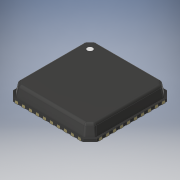
# Autodesk Inventor part: Semiconductor_QFN24-4x4
Saved by Autodesk Inventor 2018 (Build 220112000, 112)
## iProperties
Created: 2016-07-11
Part Number: Semiconductor_QFN24-4x4
Material: ABS Plastic
Document SubType Name: Modeling
Designer: Bradley
Density: 1.06 g/cm^3
Appearance: Smooth - Black
Author: Bradley
Autodesk Inventor part; units mm, degrees
ref_plane "YZ Plane" through (0, 0, 0) normal (1, 0, 0) x (0, 1, 0)
ref_plane "XZ Plane" through (0, 0, 0) normal (0, 1, 0) x (-1, 0, 0)
ref_plane "XY Plane" through (0, 0, 0) normal (0, 0, 1) x (1, 0, 0)
sketch "Sketch1" plane through (0, 0, 0) normal (0, 1, 0) x (-1, 0, 0)
  line L0 (-2.5, 3) -> (2.5, 3)
  line L1 (3, 2.5) -> (3, -2.5)
  line L2 (2.5, -3) -> (-2.5, -3)
  line L3 (-3, -2.5) -> (-3, 2.5)
  line L4 (-3, 3) -> (3, -3) construction
  line L5 (3, 3) -> (-3, -3) construction
  line L6 (3, 2.5) -> (2.5, 3)
  line L7 (-2.5, 3) -> (-3, 2.5)
  line L8 (-3, -2.5) -> (-2.5, -3)
  line L9 (2.5, -3) -> (3, -2.5)
  point P0 (0, 0)
  dimension "d0" = 6
  dimension "d1" = 6
  dimension "d68" = 0.5
  constraints: 20 end point, 8 point on line, 7 perpendicular, 2 midpoint, 2 parallel, 1 horizontal, 1 horizontal alignment
  measures "d0" distance of L4.end L5.end
  measures "d1" distance of L5.start L4.end
  measures "d68" distance of L1.start L5.start
extrude "Extrusion1" add sketch "Sketch1" along normal mid plane 0.2
sketch "Sketch2" plane through (0, -0.1, 0) normal (0, -1, 0) x (1, 0, 0)
  line L0 (2.05, 2.05) -> (-2.05, 2.05)
  line L1 (-2.05, 2.05) -> (-2.05, -2.05)
  line L2 (-2.05, -2.05) -> (2.05, -2.05)
  line L3 (2.05, -2.05) -> (2.05, 2.05)
  line L4 (2.05, 2.05) -> (-2.05, -2.05) construction
  line L5 (-2.05, 2.05) -> (2.05, -2.05) construction
  line L6 (2.5, 3) -> (-2.5, 3) projected
  line L7 (-3, 2.5) -> (-3, -2.5) projected
  line L8 (-2.5, -3) -> (2.5, -3) projected
  line L9 (3, -2.5) -> (3, 2.5) projected
  line L10 (2.375, -3) -> (2.125, -3)
  line L11 (2.125, -3) -> (2.125, -2.6)
  line L12 (2.125, -2.6) -> (2.375, -2.6)
  line L13 (2.375, -2.6) -> (2.375, -3)
  line L14 (3, -2.375) -> (2.6, -2.375)
  line L15 (2.6, -2.375) -> (2.6, -2.125)
  line L16 (2.6, -2.125) -> (3, -2.125)
  line L17 (3, -2.125) -> (3, -2.375)
  line L18 (2.375, 3) -> (2.125, 3)
  line L19 (2.125, 3) -> (2.125, 2.6)
  line L20 (2.125, 2.6) -> (2.375, 2.6)
  line L21 (2.375, 2.6) -> (2.375, 3)
  line L22 (-3, -2.375) -> (-2.6, -2.375)
  line L23 (-2.6, -2.375) -> (-2.6, -2.125)
  line L24 (-2.6, -2.125) -> (-3, -2.125)
  line L25 (-3, -2.125) -> (-3, -2.375)
  line L26 (3, -1.875) -> (2.6, -1.875)
  line L27 (2.6, -1.875) -> (2.6, -1.625)
  line L28 (2.6, -1.625) -> (3, -1.625)
  line L29 (3, -1.625) -> (3, -1.875)
  line L30 (-3, -1.875) -> (-2.6, -1.875)
  line L31 (-3, -1.625) -> (-3, -1.875)
  line L32 (-2.6, -1.625) -> (-3, -1.625)
  line L33 (-2.6, -1.875) -> (-2.6, -1.625)
  line L34 (3, -1.375) -> (2.6, -1.375)
  line L35 (2.6, -1.375) -> (2.6, -1.125)
  line L36 (2.6, -1.125) -> (3, -1.125)
  line L37 (3, -1.125) -> (3, -1.375)
  line L38 (-3, -1.375) -> (-2.6, -1.375)
  line L39 (-3, -1.125) -> (-3, -1.375)
  line L40 (-2.6, -1.125) -> (-3, -1.125)
  line L41 (-2.6, -1.375) -> (-2.6, -1.125)
  line L42 (3, -0.875) -> (2.6, -0.875)
  line L43 (2.6, -0.875) -> (2.6, -0.625)
  line L44 (2.6, -0.625) -> (3, -0.625)
  line L45 (3, -0.625) -> (3, -0.875)
  line L46 (-3, -0.875) -> (-2.6, -0.875)
  line L47 (-3, -0.625) -> (-3, -0.875)
  line L48 (-2.6, -0.625) -> (-3, -0.625)
  line L49 (-2.6, -0.875) -> (-2.6, -0.625)
  line L50 (3, -0.375) -> (2.6, -0.375)
  line L51 (2.6, -0.375) -> (2.6, -0.125)
  line L52 (2.6, -0.125) -> (3, -0.125)
  line L53 (3, -0.125) -> (3, -0.375)
  line L54 (-3, -0.375) -> (-2.6, -0.375)
  line L55 (-3, -0.125) -> (-3, -0.375)
  line L56 (-2.6, -0.125) -> (-3, -0.125)
  line L57 (-2.6, -0.375) -> (-2.6, -0.125)
  line L58 (1.875, -3) -> (1.625, -3)
  line L59 (1.625, -3) -> (1.625, -2.6)
  line L60 (1.625, -2.6) -> (1.875, -2.6)
  line L61 (1.875, -2.6) -> (1.875, -3)
  line L62 (1.625, 2.6) -> (1.875, 2.6)
  line L63 (1.625, 3) -> (1.625, 2.6)
  line L64 (1.875, 3) -> (1.625, 3)
  line L65 (1.875, 2.6) -> (1.875, 3)
  line L66 (1.375, -3) -> (1.125, -3)
  line L67 (1.125, -3) -> (1.125, -2.6)
  line L68 (1.125, -2.6) -> (1.375, -2.6)
  line L69 (1.375, -2.6) -> (1.375, -3)
  line L70 (1.125, 2.6) -> (1.375, 2.6)
  line L71 (1.125, 3) -> (1.125, 2.6)
  line L72 (1.375, 3) -> (1.125, 3)
  line L73 (1.375, 2.6) -> (1.375, 3)
  line L74 (0.875, -3) -> (0.625, -3)
  line L75 (0.625, -3) -> (0.625, -2.6)
  line L76 (0.625, -2.6) -> (0.875, -2.6)
  line L77 (0.875, -2.6) -> (0.875, -3)
  line L78 (0.625, 2.6) -> (0.875, 2.6)
  line L79 (0.625, 3) -> (0.625, 2.6)
  line L80 (0.875, 3) -> (0.625, 3)
  line L81 (0.875, 2.6) -> (0.875, 3)
  line L82 (0.375, -3) -> (0.125, -3)
  line L83 (0.125, -3) -> (0.125, -2.6)
  line L84 (0.125, -2.6) -> (0.375, -2.6)
  line L85 (0.375, -2.6) -> (0.375, -3)
  line L86 (0.125, 2.6) -> (0.375, 2.6)
  line L87 (0.125, 3) -> (0.125, 2.6)
  line L88 (0.375, 3) -> (0.125, 3)
  line L89 (0.375, 2.6) -> (0.375, 3)
  line L90 (-2.5, 3) -> (-3, 2.5) projected
  line L91 (-3, -2.5) -> (-2.5, -3) projected
  line L92 (2.5, -3) -> (3, -2.5) projected
  line L93 (3, 2.5) -> (2.5, 3) projected
  line L94 (3, 0.125) -> (2.6, 0.125)
  line L95 (2.6, 0.125) -> (2.6, 0.375)
  line L96 (2.6, 0.375) -> (3, 0.375)
  line L97 (3, 0.375) -> (3, 0.125)
  line L98 (-3, 0.125) -> (-2.6, 0.125)
  line L99 (-3, 0.375) -> (-3, 0.125)
  line L100 (-2.6, 0.375) -> (-3, 0.375)
  line L101 (-2.6, 0.125) -> (-2.6, 0.375)
  line L102 (3, 0.625) -> (2.6, 0.625)
  line L103 (2.6, 0.625) -> (2.6, 0.875)
  line L104 (2.6, 0.875) -> (3, 0.875)
  line L105 (3, 0.875) -> (3, 0.625)
  line L106 (-3, 0.625) -> (-2.6, 0.625)
  line L107 (-3, 0.875) -> (-3, 0.625)
  line L108 (-2.6, 0.875) -> (-3, 0.875)
  line L109 (-2.6, 0.625) -> (-2.6, 0.875)
  line L110 (3, 1.125) -> (2.6, 1.125)
  line L111 (2.6, 1.125) -> (2.6, 1.375)
  line L112 (2.6, 1.375) -> (3, 1.375)
  line L113 (3, 1.375) -> (3, 1.125)
  line L114 (-3, 1.125) -> (-2.6, 1.125)
  line L115 (-3, 1.375) -> (-3, 1.125)
  line L116 (-2.6, 1.375) -> (-3, 1.375)
  line L117 (-2.6, 1.125) -> (-2.6, 1.375)
  line L118 (3, 1.625) -> (2.6, 1.625)
  line L119 (2.6, 1.625) -> (2.6, 1.875)
  line L120 (2.6, 1.875) -> (3, 1.875)
  line L121 (3, 1.875) -> (3, 1.625)
  line L122 (-3, 1.625) -> (-2.6, 1.625)
  line L123 (-3, 1.875) -> (-3, 1.625)
  line L124 (-2.6, 1.875) -> (-3, 1.875)
  line L125 (-2.6, 1.625) -> (-2.6, 1.875)
  line L126 (3, 2.125) -> (2.6, 2.125)
  line L127 (2.6, 2.125) -> (2.6, 2.375)
  line L128 (2.6, 2.375) -> (3, 2.375)
  line L129 (3, 2.375) -> (3, 2.125)
  line L130 (-3, 2.125) -> (-2.6, 2.125)
  line L131 (-3, 2.375) -> (-3, 2.125)
  line L132 (-2.6, 2.375) -> (-3, 2.375)
  line L133 (-2.6, 2.125) -> (-2.6, 2.375)
  line L134 (-0.125, -3) -> (-0.375, -3)
  line L135 (-0.375, -3) -> (-0.375, -2.6)
  line L136 (-0.375, -2.6) -> (-0.125, -2.6)
  line L137 (-0.125, -2.6) -> (-0.125, -3)
  line L138 (-0.375, 2.6) -> (-0.125, 2.6)
  line L139 (-0.375, 3) -> (-0.375, 2.6)
  line L140 (-0.125, 3) -> (-0.375, 3)
  line L141 (-0.125, 2.6) -> (-0.125, 3)
  line L142 (-0.625, -3) -> (-0.875, -3)
  line L143 (-0.875, -3) -> (-0.875, -2.6)
  line L144 (-0.875, -2.6) -> (-0.625, -2.6)
  line L145 (-0.625, -2.6) -> (-0.625, -3)
  line L146 (-0.875, 2.6) -> (-0.625, 2.6)
  line L147 (-0.875, 3) -> (-0.875, 2.6)
  line L148 (-0.625, 3) -> (-0.875, 3)
  line L149 (-0.625, 2.6) -> (-0.625, 3)
  line L150 (-1.125, -3) -> (-1.375, -3)
  line L151 (-1.375, -3) -> (-1.375, -2.6)
  line L152 (-1.375, -2.6) -> (-1.125, -2.6)
  line L153 (-1.125, -2.6) -> (-1.125, -3)
  line L154 (-1.375, 2.6) -> (-1.125, 2.6)
  line L155 (-1.375, 3) -> (-1.375, 2.6)
  line L156 (-1.125, 3) -> (-1.375, 3)
  line L157 (-1.125, 2.6) -> (-1.125, 3)
  line L158 (-1.625, -3) -> (-1.875, -3)
  line L159 (-1.875, -3) -> (-1.875, -2.6)
  line L160 (-1.875, -2.6) -> (-1.625, -2.6)
  line L161 (-1.625, -2.6) -> (-1.625, -3)
  line L162 (-1.875, 2.6) -> (-1.625, 2.6)
  line L163 (-1.875, 3) -> (-1.875, 2.6)
  line L164 (-1.625, 3) -> (-1.875, 3)
  line L165 (-1.625, 2.6) -> (-1.625, 3)
  line L166 (-2.125, -3) -> (-2.375, -3)
  line L167 (-2.375, -3) -> (-2.375, -2.6)
  line L168 (-2.375, -2.6) -> (-2.125, -2.6)
  line L169 (-2.125, -2.6) -> (-2.125, -3)
  line L170 (-2.375, 2.6) -> (-2.125, 2.6)
  line L171 (-2.375, 3) -> (-2.375, 2.6)
  line L172 (-2.125, 3) -> (-2.375, 3)
  line L173 (-2.125, 2.6) -> (-2.125, 3)
  point P0 (0, 0)
  point P1 (0.25, -2.6)
  point P2 (-2.6, -0.25)
  point P3 (-2.6, -0.75)
  point P4 (1.25, -2.6)
  point P5 (0, 0)
  point P6 (0, 0)
  dimension "d4" = 4.1
  dimension "d5" = 4.1
  dimension "d8" = 0.4
  dimension "d9" = 0.25
  dimension "d20" = 0.5
  dimension "d63" = 0.5
  dimension "d76" = 0.25
  dimension "d77" = 0.25
  constraints: 332 end point, 10 parallel, 8 midpoint, 6 equal length, 6 horizontal, 6 point on line, 5 perpendicular, 2 collinear, 1 vertical, 288 other
  measures "d4" distance of L4.end L2.end
  measures "d5" distance of L2.end L0.start
  measures "d8" distance of L14.start L14.end
  measures "d9" distance of L14.end L15.end
  measures "d20" distance of L14.start L26.start
  measures "d63" distance of L10.start L58.start
  measures "d76" vertical distance of point (0, 0) point (-2.6, -0.25)
  measures "d77" horizontal distance of point (0, 0) point (0.25, -2.6)
extrude "Extrusion2" add sketch "Sketch2" along normal blind 0.02 contours L3 L2 L1 L0 | L21 L20 L19 L6 | L9 L126 L127 L128 | L65 L62 L63 L6 | L9 L118 L119 L120 | L73 L70 L71 L6 | L9 L110 L111 L112 | L81 L78 L79 L6 | L9 L102 L103 L104 | L89 L86 L87 L6 | L9 L94 L95 L96 | L141 L138 L139 L6 | L9 L50 L51 L52 | L149 L146 L147 L6 | L9 L42 L43 L44 | L157 L154 L155 L6 | L9 L34 L35 L36 | L165 L162 L163 L6 | L9 L26 L27 L28 | L173 L170 L171 L6 | L9 L14 L15 L16 | L132 L133 L130 L7 | L8 L11 L12 L13 | L124 L125 L122 L7 | L8 L59 L60 L61 | L116 L117 L114 L7 | L8 L67 L68 L69 | L108 L109 L106 L7 | L8 L75 L76 L77 | L100 L101 L98 L7 | L8 L83 L84 L85 | L56 L57 L54 L7 | L8 L135 L136 L137 | L48 L49 L46 L7 | L8 L143 L144 L145 | L40 L41 L38 L7 | L8 L151 L152 L153 | L32 L33 L30 L7 | L8 L159 L160 L161 | L24 L23 L22 L7 | L8 L167 L168 L169
sketch "Sketch3" plane through (-3, -0.1, 3) normal (-1, 0, 0) x (0, 0, 1)
  line L0 (-5.5, 0.2) -> (-0.5, 0.2) projected
  line L1 (-0.875, 0) -> (-1.125, 0) projected
  line L2 (-5.375, 0) -> (-5.375, -0.02) projected
  line L3 (-5.125, -0.02) -> (-5.375, -0.02) projected
  line L4 (-5.125, 0) -> (-5.125, -0.02) projected
  line L5 (-4.875, 0) -> (-5.125, 0) projected
  line L6 (-4.875, 0) -> (-4.875, -0.02) projected
  line L7 (-4.625, -0.02) -> (-4.875, -0.02) projected
  line L8 (-4.625, 0) -> (-4.625, -0.02) projected
  line L9 (-4.375, 0) -> (-4.625, 0) projected
  line L10 (-4.375, 0) -> (-4.375, -0.02) projected
  line L11 (-4.125, -0.02) -> (-4.375, -0.02) projected
  line L12 (-4.125, 0) -> (-4.125, -0.02) projected
  line L13 (-3.875, 0) -> (-4.125, 0) projected
  line L14 (-3.875, 0) -> (-3.875, -0.02) projected
  line L15 (-3.625, -0.02) -> (-3.875, -0.02) projected
  line L16 (-3.625, 0) -> (-3.625, -0.02) projected
  line L17 (-3.375, 0) -> (-3.625, 0) projected
  line L18 (-3.375, 0) -> (-3.375, -0.02) projected
  line L19 (-3.125, -0.02) -> (-3.375, -0.02) projected
  line L20 (-3.125, 0) -> (-3.125, -0.02) projected
  line L21 (-1.375, 0) -> (-1.625, 0) projected
  line L22 (-5.375, 0) -> (-5.125, 0) projected
  line L23 (-5.375, 0) -> (-5.3594, 0.183)
  line L24 (-5.3594, 0.183) -> (-5.1406, 0.183)
  line L25 (-5.1406, 0.183) -> (-5.125, 0)
  line L26 (-0.5, 0.2) -> (-0.5, 0) projected
  line L27 (-5.5, 0) -> (-5.5, 0.2) projected
  line L28 (-5.375, 0) -> (-5.5, 0) projected
  line L29 (-2.875, 0) -> (-3.125, 0) projected
  line L30 (-2.875, 0) -> (-2.875, -0.02) projected
  line L31 (-2.625, -0.02) -> (-2.875, -0.02) projected
  line L32 (-2.625, 0) -> (-2.625, -0.02) projected
  line L33 (-2.375, 0) -> (-2.625, 0) projected
  line L34 (-2.375, 0) -> (-2.375, -0.02) projected
  line L35 (-2.125, -0.02) -> (-2.375, -0.02) projected
  line L36 (-2.125, 0) -> (-2.125, -0.02) projected
  line L37 (-1.875, 0) -> (-2.125, 0) projected
  line L38 (-1.875, 0) -> (-1.875, -0.02) projected
  line L39 (-1.625, -0.02) -> (-1.875, -0.02) projected
  line L40 (-1.625, 0) -> (-1.625, -0.02) projected
  line L41 (-1.375, 0) -> (-1.375, -0.02) projected
  line L42 (-1.125, -0.02) -> (-1.375, -0.02) projected
  line L43 (-1.125, 0) -> (-1.125, -0.02) projected
  line L44 (-0.875, 0) -> (-0.875, -0.02) projected
  line L45 (-0.625, -0.02) -> (-0.875, -0.02) projected
  line L46 (-0.625, 0) -> (-0.625, -0.02) projected
  line L47 (-0.5, 0) -> (-0.625, 0) projected
  point P0 (-3, 0.1)
  dimension "d28" = 0.203
  dimension "d29" = 0.25
  dimension "d30" = 0.2188
  constraints: 6 end point, 1 equal length, 1 parallel
  measures "d28" distance between parallel lines of L3 L24
  measures "d29" distance of L3.start L2.end
  measures "d30" distance of L23.end L24.end
extrude "Extrusion3" add sketch "Sketch3" along normal blind 0.01 contours L22 L4 L3 L2 | L23 L24 L25 L22
pattern_linear "Rectangular Pattern1" count 10 spacing 0.5 along (0, 0, 1) of "Extrusion3"
pattern_circular "Circular Pattern1" count 4 over 360 about axis through (0, -10, 0) along (0, 1, 0) of "Extrusion3", "Rectangular Pattern1"
sketch "Sketch6" plane through (0, 0.1, 0) normal (0, 1, 0) x (1, 0, 0)
  line L0 (-3, -2.5) -> (-2.5, -3) projected
  line L1 (-2.5, -3) -> (2.5, -3) projected
  line L2 (2.5, -3) -> (3, -2.5) projected
  line L3 (3, -2.5) -> (3, 2.5) projected
  line L4 (3, 2.5) -> (2.5, 3) projected
  line L5 (2.5, 3) -> (-2.5, 3) projected
  line L6 (-2.5, 3) -> (-3, 2.5) projected
  line L7 (-3, 2.5) -> (-3, -2.5) projected
  line L8 (2.4482, 2.875) -> (2.875, 2.4482)
  line L9 (2.875, 2.4482) -> (2.875, -2.4482)
  line L10 (2.875, -2.4482) -> (2.4482, -2.875)
  line L11 (2.4482, -2.875) -> (-2.4482, -2.875)
  line L12 (-2.4482, -2.875) -> (-2.875, -2.4482)
  line L13 (-2.875, -2.4482) -> (-2.875, 2.4482)
  line L14 (-2.875, 2.4482) -> (-2.4482, 2.875)
  line L15 (-2.4482, 2.875) -> (2.4482, 2.875)
  point P0 (0, 0)
  dimension "d78" = 5.75
  constraints: 16 end point, 7 other
  measures "d78" distance between parallel lines of L13 L9
extrude "Extrusion6" add sketch "Sketch6" along normal blind 0.75 draft -12 contours L8 L9 L10 L11 L12 L13 L14 L15
fillet "Fillet1" radius 0.2 16 edges at (2.7156, 0.85, 0) (2.7953, 0.475, 2.4152) (2.7953, 0.475, -2.4152) (2.5489, 0.85, 2.5489) (2.4152, 0.475, 2.7953) (0, 0.85, 2.7156) (-2.4152, 0.475, 2.7953) (-2.5489, 0.85, 2.5489) (-2.7953, 0.475, 2.4152) (-2.7156, 0.85, 0) (-2.7953, 0.475, -2.4152) (-2.5489, 0.85, -2.5489) (-2.4152, 0.475, -2.7953) (0, 0.85, -2.7156) (2.4152, 0.475, -2.7953) (2.5489, 0.85, -2.5489)
sketch "Sketch7" plane through (0, 0.85, 0) normal (0, 1, 0) x (1, 0, 0)
  circle A0 centre (-2.0536, 2.0536) radius 0.2
  line L0 (-2.5536, -2.3151) -> (-2.5536, 2.3151) projected
  line L1 (-2.3151, -2.5536) -> (-2.5536, -2.3151) projected
  line L2 (2.3151, -2.5536) -> (-2.3151, -2.5536) projected
  line L3 (2.5536, -2.3151) -> (2.3151, -2.5536) projected
  line L4 (2.5536, 2.3151) -> (2.5536, -2.3151) projected
  line L5 (2.3151, 2.5536) -> (2.5536, 2.3151) projected
  line L6 (-2.3151, 2.5536) -> (2.3151, 2.5536) projected
  line L7 (-2.5536, 2.3151) -> (-2.3151, 2.5536) projected
  circle A1 centre (-2.0536, 2.0536) radius 0.5 construction
  line L8 (-2.3151, 2.5536) -> (2.3151, 2.5536) construction
  line L9 (-2.5536, -2.3151) -> (-2.5536, 2.3151) construction
  point P0 (0, 0)
  dimension "d82" = 0.4
  dimension "d83" = 0.3
  constraints: 2 centre point, 2 tangent, 1 coincident
  measures "d82" diameter of A0
  measures "d83" radial gap between concentric circles of A0 A1
extrude "Extrusion7" add sketch "Sketch7" along normal blind 0.01 contours A0
equation "\"d76\" = 0.5 * d20"
equation "\"d77\" = d76"
equation "\"d30\" = 0.875 * d29"
body "Solid1"
